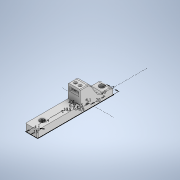
# Autodesk Inventor part: Horizontal_1_v2
Saved by Autodesk Inventor 2020.3 (Build 243373000, 373)
## iProperties
Created: 2021-03-28
Part Number: Horizontal_1_v2
Material: Generic
Document SubType Name: Modeling
Designer: sanyi
Density: 1 g/cm^3
Appearance: Default
Author: sanyi
Autodesk Inventor part; units mm, degrees
ref_plane "YZ Plane" through (0, 0, 0) normal (1, 0, 0) x (0, 1, 0)
ref_plane "XZ Plane" through (0, 0, 0) normal (0, 1, 0) x (-1, 0, 0)
ref_plane "XY Plane" through (0, 0, 0) normal (0, 0, 1) x (1, 0, 0)
sketch "Sketch1" plane through (0, 0, 0) normal (0, 1, 0) x (-1, 0, 0)
  line L0 (8.5, 19) -> (-8.5, 19)
  line L1 (-8.5, 19) -> (-8.5, -28)
  line L2 (-8.5, -28) -> (8.5, -28)
  line L3 (8.5, -28) -> (8.5, 19)
  line L4 (35.537, 0) -> (-37.6285, 0) construction
  line L5 (0, 76.31) -> (0, -83.8259) construction
  circle A0 centre (0, -20) radius 2.05
  circle A1 centre (0, 0) radius 2.05
  line L6 (6.5, 19) -> (6.5, 12.5)
  line L7 (6.5, 12.5) -> (-6.5, 12.5) construction
  line L8 (-6.5, 12.5) -> (-6.5, 19)
  line L9 (5.2605, 14) -> (-5.0586, 14) construction
  circle A2 centre (-3.25, 14) radius 1.05
  circle A3 centre (3.25, 14) radius 1.05
  line L10 (6.5, 12.5) -> (6.5, 8.5)
  line L11 (6.5, 8.5) -> (-6.5, 8.5) construction
  line L12 (-6.5, 8.5) -> (-6.5, 12.5)
  circle A4 centre (0, 8.5) radius 2.5
  line L13 (6.5, 8.5) -> (0.9615, 6.1923)
  line L14 (-0.9615, 6.1923) -> (-6.5, 8.5)
  line L15 (6.5, 8.5) -> (8.5, 8.5)
  line L16 (8.5, 19) -> (8.5, 79.4)
  line L17 (8.5, 79.4) -> (-8.5, 79.4)
  line L18 (-8.5, 79.4) -> (-8.5, 19)
  circle A5 centre (0, 64.4) radius 2.05
  line L19 (8.5, 30.5) -> (-8.5, 30.5) construction
  line L20 (8.5, 25) -> (-8.5, 25) construction
  circle A6 centre (3.25, 14) radius 1.5
  circle A7 centre (-3.25, 14) radius 1.5
  circle A8 centre (3.25, 14) radius 2.45
  circle A9 centre (-3.25, 14) radius 2.45
  dimension "d0" = 17
  dimension "d1" = 20
  dimension "d2" = 4.1
  dimension "d3" = 8
  dimension "d4" = 19
  dimension "d7" = 13
  dimension "d8" = 6.5
  dimension "d11" = 1.5
  dimension "d12" = 6.5
  dimension "d13" = 4
  dimension "d14" = 5
  dimension "d76" = 4.1
  dimension "d79" = 16.5
  dimension "d80" = 11
  dimension "d81" = 54.4
  dimension "d82" = 15
  dimension "d89" = 3
  dimension "d90" = 4.9
  dimension "d91" = 2.1
  constraints: 42 end point, 15 point on line, 10 centre point, 7 parallel, 7 perpendicular, 4 coincident, 4 equal radius, 2 collinear, 2 horizontal, 2 point on circle, 2 tangent, 1 midpoint, 1 symmetric about line, 1 vertical, 2 other
  measures "d0" distance of L1.end L2.end
  measures "d1" distance of A0.centre point (0, 0)
  measures "d2" diameter of A1
  measures "d3" distance from line of L2 A0.centre
  measures "d4" distance from line of L0 point (0, 0)
  measures "d7" distance of L6.end L7.end
  measures "d8" distance of L6.start L6.end
  measures "d11" distance between parallel lines of L7 L9
  measures "d12" distance of A2.centre A3.centre
  measures "d13" distance between parallel lines of L7 L11
  measures "d14" diameter of A4
  measures "d76" diameter of A5
  measures "d79" distance from line of L19 A3.centre
  measures "d80" distance from line of A3.centre L20
  measures "d81" distance between parallel lines of L17 L20
  measures "d82" distance from line of L17 A5.centre
  measures "d89" diameter of A6
  measures "d90" diameter of A8
  measures "d91" diameter of A3
extrude "Extrusion1" add sketch "Sketch1" along normal blind 20 contours L6 L10 L13 A4 L14 L12 L8 L0 | A2 | A3 | A6 | A7 | A8 | A9
extrude "Extrusion2" add sketch "Sketch1" along normal blind 25.8 contours L3 L15 L10 L6 L0 | L3 L2 L1 L0 L8 L12 L14 A4 L13 L15
sketch "Sketch3" plane through (0, 20, 0) normal (0, 1, 0) x (1, 0, 0)
  circle A0 centre (3.25, -14) radius 1.05 projected
  circle A1 centre (-3.25, -14) radius 1.05 projected
  point P0 (0, 0)
extrude "Extrusion4" cut sketch "Sketch3" against normal up to surface (20 mm away)
extrude "Extrusion15" cut sketch "Sketch1" along normal blind 11.4 contours A2 | A3 | A6 | A7
extrude "Extrusion16" cut sketch "Sketch1" along normal blind 7.3 contours A8 | A9
sketch "Sketch5" plane through (0, 25.8, 0) normal (0, 1, 0) x (1, 0, 0)
  circle A0 centre (0, 0) radius 2.05 projected
  circle A1 centre (0, 20) radius 2.05 projected
  circle A2 centre (0, 0) radius 3.75
  circle A3 centre (0, 20) radius 3.75
  dimension "d29" = 7.5
  dimension "d30" = 7.5
  constraints: 2 centre point, 2 coincident
  measures "d29" diameter of A2
  measures "d30" diameter of A3
extrude "Extrusion6" cut sketch "Sketch5" against normal blind 20.8
sketch "Sketch6" plane through (0, 25.8, 0) normal (0, 1, 0) x (1, 0, 0)
  circle A0 centre (0, 0) radius 3.75 projected
  circle A1 centre (0, 20) radius 3.75 projected
  circle A2 centre (0, 20) radius 3.75 projected
  circle A3 centre (0, 0) radius 3.75 projected
  line L0 (-8.5, -19) -> (-6.5, -19) projected
  line L1 (-6.5, -8.5) -> (-0.9615, -6.1923) projected
  arc A4 (0.9615, -6.1923) -> (-0.9615, -6.1923) centre (0, -8.5) ccw projected
  line L2 (0.9615, -6.1923) -> (6.5, -8.5) projected
  line L3 (6.5, -8.5) -> (6.5, -19) projected
  line L4 (8.5, -19) -> (8.5, 28) projected
  line L5 (8.5, 28) -> (-8.5, 28) projected
  line L6 (-8.5, 28) -> (-8.5, -19) projected
  line L7 (-8.5, 7) -> (8.5, 7)
  line L8 (-6.5, -19) -> (-6.5, -8.5) projected
  line L9 (6.5, -19) -> (8.5, -19) projected
  dimension "d41" = 13
  constraints: 2 end point, 1 coincident, 1 perpendicular, 1 point on line
  measures "d41" distance from line of A1.centre L7
extrude "Extrusion7" cut sketch "Sketch6" against normal blind 15.8 contours L6 L5 L4 L7
extrude "Extrusion13" add sketch "Sketch1" along normal blind 10 contours L0 L18 L17 L16
chamfer "Chamfer2" distance 10 distance2 15.8 1 edges at (0, 25.8, -7) measured on face at (0, 25.8, -6.5)
sketch "Sketch11" plane through (0, 10, 0) normal (0, 1, 0) x (1, 0, 0)
  circle A0 centre (0, -64.4) radius 2.05 projected
  circle A1 centre (0, -64.4) radius 3.75
  point P0 (0, 0)
  dimension "d85" = 7.5
  constraints: 1 centre point, 1 coincident
  measures "d85" diameter of A1
extrude "Extrusion14" cut sketch "Sketch11" against normal blind 5
ref_plane "Work Plane1" through (-6.5, 0, 8.5) normal (0, -0.4226183, 0.9063078) x (1, 0, 0)
sketch "Sketch9" plane through (0, 25.8, 0) normal (0, 1, 0) x (1, 0, 0)
  line L0 (2.25, -3) -> (8.5, -3) projected
  arc A0 (-2.25, -3) -> (2.25, -3) centre (0, 0) ccw projected
  line L1 (-8.5, -3) -> (-2.25, -3) projected
  line L2 (-8.5, -3) -> (-8.5, -19) projected
  line L3 (-6.5, -8.5) -> (-0.9615, -6.1923) projected
  arc A1 (0.9615, -6.1923) -> (-0.9615, -6.1923) centre (0, -8.5) ccw projected
  line L4 (0.9615, -6.1923) -> (6.5, -8.5) projected
  line L5 (6.5, -8.5) -> (6.5, -19) projected
  line L6 (6.5, -19) -> (8.5, -19) projected
  line L7 (8.5, -19) -> (8.5, -3) projected
  circle A2 centre (3.25, -14) radius 1.05 projected
  circle A3 centre (-3.25, -14) radius 1.05 projected
  line L8 (6.5, -8.5) -> (0.9615, -6.1923) projected
  arc A4 (-0.9615, -6.1923) -> (0.9615, -6.1923) centre (0, -8.5) ccw projected
  line L9 (-0.9615, -6.1923) -> (-6.5, -8.5) projected
  line L10 (-6.5, -19) -> (6.5, -19) projected
  line L11 (6.5, -19) -> (6.5, -8.5) projected
  line L12 (-6.5, -8.5) -> (-6.5, -19) projected
  line L13 (-8.5, -19) -> (-6.5, -19) projected
  line L14 (-6.5, -19) -> (-6.5, -8.5) projected
sketch "Sketch7" plane through (-6.5, 0, 8.5) normal (0, -0.4226183, 0.9063078) x (1, 0, 0)
  circle A0 centre (6.5, 1) radius 2.5
  line L0 (0, 0) -> (13, 0) projected
  line L1 (6.5, -2.449) -> (6.5, 4.9828)
  line L2 (9, -4.085) -> (4, -4.085)
  line L3 (4, -4.085) -> (4, 1)
  line L4 (4, 1) -> (9, 1)
  line L5 (9, 1) -> (9, -4.085)
  point P0 (6.5, 0)
  point P1 (6.5, 0)
  dimension "d47" = 5
  dimension "d50" = 1
  constraints: 10 end point, 2 parallel, 2 perpendicular, 2 point on circle, 2 point on line, 1 centre point, 1 horizontal, 1 midpoint, 1 tangent
  measures "d47" diameter of A0
  measures "d50" distance of point (6.5, 0) A0.centre
extrude "Extrusion8" cut sketch "Sketch7" along normal blind 10
fillet "Fillet4" radius 2 1 edges at (0, 2.6961, 11)
extrude "Extrusion10" add sketch "Sketch9" along normal blind 3.5 contours L0 L7 L6 L5 L4 A1 L3 L12 L13 L2 L1 A0 | L10 L12 L3 A4 L4 L5 | A4 A1 | A2 | A3
chamfer "Chamfer5" distance 3.5 angle 45 2 edges at (5.375, 29.3, 3) (-5.375, 29.3, 3)
sketch "Sketch10" plane through (0, 29.3, 0) normal (0, 1, 0) x (1, 0, 0)
  circle A0 centre (-3.25, -14) radius 1.05 projected
  circle A1 centre (3.25, -14) radius 1.05 projected
  circle A2 centre (-3.25, -14) radius 1.05
  circle A3 centre (3.25, -14) radius 1.05
  circle A4 centre (-3.25, -14) radius 2.15
  circle A5 centre (3.25, -14) radius 2.15
  point P0 (0, 0)
  dimension "d63" = 2.1
  dimension "d65" = 4.3
  dimension "d66" = 4.3
  constraints: 4 centre point, 4 coincident, 1 equal radius
  measures "d63" diameter of A2
  measures "d65" diameter of A4
  measures "d66" diameter of A5
extrude "Extrusion11" cut sketch "Sketch10" against normal up to surface (3.5 mm away) contours A0 | A1
extrude "Extrusion12" cut sketch "Sketch10" against normal blind 2
fillet "Fillet6" radius 10 1 edges at (0, 10, -7)
fillet "Fillet6" radius 5 1 edges at (0, 10, -28)
fillet "Fillet6" radius 5 2 edges at (5.375, 25.8, 3) (-5.375, 25.8, 3)
fillet "Fillet6" radius 5 1 edges at (0, 29.3, 6.5)
fillet "Fillet7" radius 1 20 edges at (8.5, 28.9194, 6.6577) (8.5, 27.014, 4.214) (8.5, 25.7808, 3.024) (8.5, 19.9915, -0.6763) (8.5, 11.2399, -7.6826) (8.5, 10, -17.7527) (8.5, 8.5355, -26.5355) (8.5, 2.5, -28) (8.5, 29.3, 13.7855) (-8.5, 28.9194, 6.6577) (-8.5, 27.014, 4.214) (-8.5, 25.7808, 3.024) (-8.5, 19.9915, -0.6763) (-8.5, 11.2399, -7.6826) (-8.5, 10, -17.7527) (-8.5, 8.5355, -26.5355) (-8.5, 2.5, -28) (-8.5, 29.3, 13.7855) (8.5, 5, 79.4) (-8.5, 5, 79.4)
body "Solid1"
